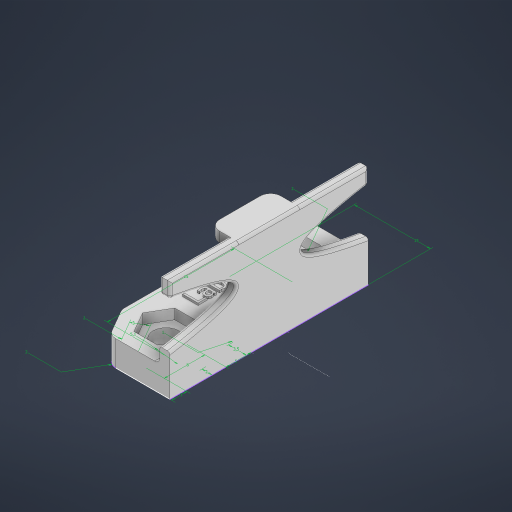
# Autodesk Inventor part: soporte_pinzas_abiertas
Saved by Autodesk Inventor 2024.1 (Build 281209000, 209)
## iProperties
Created: 2023-06-27
Part Number: soporte_pinzas_abiertas
Material: Generic
Document SubType Name: Modeling
Designer: LabTel_Admin
Density: 1 g/cm^3
Appearance: Default
Author: LabTel_Admin
Autodesk Inventor part; units mm, degrees
ref_plane "YZ Plane" through (0, 0, 0) normal (1, 0, 0) x (0, 1, 0)
ref_plane "XZ Plane" through (0, 0, 0) normal (0, 1, 0) x (-1, 0, 0)
ref_plane "XY Plane" through (0, 0, 0) normal (0, 0, 1) x (1, 0, 0)
sketch "Sketch2" plane through (0, 0, 0) normal (0, 1, 0) x (-1, 0, 0)
  line L0 (15.1065, 12.5) -> (17.4159, 16.5)
  line L1 (17.4159, 16.5) -> (22.0347, 16.5)
  line L2 (22.0347, 16.5) -> (24.3441, 12.5)
  line L3 (24.3441, 12.5) -> (22.0347, 8.5)
  line L4 (22.0347, 8.5) -> (17.4159, 8.5)
  line L5 (17.4159, 8.5) -> (15.1065, 12.5)
  circle A0 centre (19.7253, 12.5) radius 2.55
  line L6 (11.9711, 19.5) -> (22.612, 19.5)
  line L7 (24.3441, 18.5) -> (26.7031, 14.414)
  line L8 (26.9711, 13.414) -> (26.9711, 0.8204)
  line L9 (0, 0) -> (8.2774, 0) construction
  line L10 (15.1065, -12.5) -> (17.4159, -16.5)
  line L11 (17.4159, -16.5) -> (22.0347, -16.5)
  line L12 (22.0347, -16.5) -> (24.3441, -12.5)
  line L13 (24.3441, -12.5) -> (22.0347, -8.5)
  line L14 (22.0347, -8.5) -> (17.4159, -8.5)
  line L15 (17.4159, -8.5) -> (15.1065, -12.5)
  circle A1 centre (19.7253, -12.5) radius 2.55
  line L16 (13.6603, -19.5) -> (22.612, -19.5)
  line L17 (24.3441, -18.5) -> (26.7031, -14.414)
  line L18 (26.9711, -13.414) -> (26.9711, -0.8204)
  line L19 (11.9711, -19.5) -> (13.6603, -19.5)
  line L20 (26.9711, 0.8204) -> (26.9711, -0.8204)
  arc A2 (24.3441, 18.5) -> (22.612, 19.5) centre (22.612, 17.5) ccw
  arc A3 (26.9711, 13.414) -> (26.7031, 14.414) centre (24.9711, 13.414) ccw
  arc A4 (22.612, -19.5) -> (24.3441, -18.5) centre (22.612, -17.5) ccw
  arc A5 (26.7031, -14.414) -> (26.9711, -13.414) centre (24.9711, -13.414) ccw
  line L21 (11.9711, 19.5) -> (11.9711, -19.5)
  line L22 (11.9711, 3.5) -> (15.4711, 3.5)
  line L23 (15.9711, 3.366) -> (17.1876, 2.6637)
  line L24 (17.6876, 1.7976) -> (17.6876, -1.5)
  arc A6 (15.9711, 3.366) -> (15.4711, 3.5) centre (15.4711, 2.5) ccw
  arc A7 (17.6876, 1.7976) -> (17.1876, 2.6637) centre (16.6876, 1.7976) ccw
  line L25 (11.9711, -3.5) -> (15.4711, -3.5)
  line L26 (15.9711, -3.366) -> (17.1876, -2.6637)
  line L27 (17.6876, -1.7976) -> (17.6876, -1.5)
  arc A8 (15.4711, -3.5) -> (15.9711, -3.366) centre (15.4711, -2.5) ccw
  arc A9 (17.1876, -2.6637) -> (17.6876, -1.7976) centre (16.6876, -1.7976) ccw
  line L28 (13.9711, 3.5) -> (13.9711, 19.5)
  line L29 (13.9711, -3.5) -> (13.9711, -19.5)
  point P0 (19.7253, 8.5)
  point P1 (19.7253, 16.5)
  point P2 (23.7667, 19.5)
  point P3 (26.9711, 13.9499)
  point P4 (23.1894, 14.5)
  point P5 (19.7253, -8.5)
  point P6 (19.7253, -16.5)
  point P7 (23.7667, -19.5)
  point P8 (26.9711, -13.9499)
  point P9 (23.1894, -14.5)
  point P10 (25.239, 0.1796)
  point P11 (25.239, -0.1796)
  point P12 (26.9711, -7.1172)
  point P13 (13.4711, -19.5)
  dimension "d18" = 8
  dimension "d19" = 5.1
  dimension "d21" = 3
  dimension "d22" = 3
  dimension "d27" = 25
  dimension "d35" = 2
  dimension "d36" = 2
  dimension "d37" = 2
  dimension "d49" = 5
  dimension "d50" = 1
  dimension "d51" = 3.5
  dimension "d52" = 15
  dimension "d53" = 2
  constraints: 60 end point, 24 symmetric about line, 16 point on circle, 12 tangent, 11 point on line, 10 centre point, 4 midpoint, 3 horizontal, 3 vertical, 2 coincident, 2 equal radius, 2 perpendicular, 1 parallel, 16 other
  measures "d18" distance of point (19.725, 8.5) point (19.725, 16.5)
  measures "d19" diameter of A0
  measures "d21" distance between parallel lines of L6 L1
  measures "d22" distance from line of L7 point (23.189, 14.5)
  measures "d27" distance of point (19.725, -12.5) point (19.725, 12.5)
  measures "d35" radius of A2
  measures "d36" radius of A3
  measures "d37" radius of A4
  measures "d49" distance from line of L4 L22.start
  measures "d50" radius of A6
  measures "d51" distance of L22.start L22.end
  measures "d52" distance from line of L21 point (26.971, -7.117)
  measures "d53" distance between parallel lines of L21 L28
extrude "Extrusion9" add sketch "Sketch2" along normal blind 5 contours L6 L28 L22 L21 | L6 A2 L7 A3 L8 L20 L18 A5 L17 A4 L16 L29 L25 A8 L26 A9 L27 L24 A7 L23 A6 L22 L28 | L25 L29 L16 L19 L21
extrude "Extrusion10" add sketch "Sketch2" along normal blind 3 contours L0 L1 L2 L3 L4 L5 | L15 L14 L13 L12 L11 L10
extrude "Extrusion13" add sketch "Sketch2" along normal blind 20 contours L6 L28 L22 L21 | L25 L29 L16 L19 L21
extrude "Extrusion14" add sketch "Sketch2" along normal blind 18 contours L22 A6 L23 A7 L24 L27 A9 L26 A8 L25 L21
sketch "Sketch6" plane through (-13.9711, 5, 19.5) normal (-1, 0, 0) x (0, 0, 1)
  line L0 (-19.5, -5) -> (-19.5, 29.0321) construction
  line L1 (0, 0) -> (0, 15) projected
  line L2 (-5.086, 0) -> (-1, 0) projected
  line L3 (-16, 15) -> (0, 15) projected
  line L4 (-16, 0) -> (-16, 15) projected
  line L5 (-16, 7.5) -> (-13, 7.5)
  spline S0 degree 2 poles (0, 3) (-26, 7.5) (0, 12) knots 0 0 0 1 1 1
  line L6 (0, 3) -> (0, 12)
  line L7 (-39, 0) -> (-39, 15)
  spline S1 degree 2 poles (-39, 3) (-13, 7.5) (-39, 12) knots 0 0 0 1 1 1
  line L8 (-39, 3) -> (-39, 12)
  point P0 (-26, 7.5)
  dimension "d73" = 3
  dimension "d74" = 3
  dimension "d75" = 3
  constraints: 10 end point, 5 symmetric about line, 4 point on line, 1 collinear, 1 horizontal, 1 midpoint, 1 vertical, 6 other
  measures "d73" distance from line of L2 L6.start
  measures "d74" distance from line of L3 L6.end
  measures "d75" distance of L5.start L5.end
extrude "Extrusion15" cut sketch "Sketch6" against normal blind 20 contours S0 L1 | L7 S1
fillet "Fillet3" radius 1 2 edges at (-13.9711, 5, 11.5) (-13.9711, 5, -11.5)
fillet "Fillet4" radius 0.5 4 edges at (-13.9711, 12.5, 6.5) (-11.9711, 12.4968, 6.5) (-13.9711, 12.5, -6.5) (-11.9711, 12.4968, -6.5)
fillet "Fillet5" radius 0.51 14 edges at (-13.9711, 20, 11.5) (-13.8247, 17.1486, 19.5) (-12.9711, 17, 19.5) (-12.1175, 17.1486, 19.5) (-11.9711, 18.7537, 19.5) (-13.9711, 18.7537, 19.5) (-13.9711, 20, -11.5) (-11.9711, 20, 11.5) (-11.9711, 20, -11.5) (-13.8247, 17.1486, -19.5) (-12.9711, 17, -19.5) (-12.1175, 17.1486, -19.5) (-11.9711, 18.7537, -19.5) (-13.9711, 18.7537, -19.5)
sketch "Sketch7" plane through (0, 18, 0) normal (0, 1, 0) x (1, 0, 0)
  line L0 (-17.6876, 1.7976) -> (-17.6876, -1.7976) projected
  line L1 (-11.9711, -19.5) -> (-11.9711, 19.5) projected
  line L2 (-15.6876, -6) -> (-11.9711, -6)
  line L3 (-11.9711, -6) -> (-11.9711, 6)
  line L4 (-11.9711, 6) -> (-15.6876, 6)
  line L5 (-17.6876, 4) -> (-17.6876, -4)
  arc A0 (-17.6876, -4) -> (-15.6876, -6) centre (-15.6876, -4) ccw
  arc A1 (-15.6876, 6) -> (-17.6876, 4) centre (-15.6876, 4) ccw
  point P0 (0, 0)
  point P1 (-17.6876, -6)
  point P2 (-17.6876, 0)
  point P3 (-17.6876, 0)
  point P4 (-17.6876, 0)
  point P5 (-17.6876, 0)
  point P6 (-17.6876, -1.7976)
  dimension "d82" = 6
  dimension "d83" = 12
  dimension "d84" = 2
  constraints: 8 end point, 4 point on circle, 4 tangent, 3 point on line, 2 centre point, 2 coincident, 2 midpoint, 2 parallel, 1 equal radius, 1 horizontal, 1 perpendicular
  measures "d82" distance of point (-17.688, -6) point (-17.688, 0)
  measures "d83" distance of L3.end L2.end
  measures "d84" radius of A0
extrude "Extrusion16" add sketch "Sketch7" along normal blind 2
fillet "Fillet6" radius 0.5 1 edges at (-11.9711, 20, 0)
sketch "Sketch8" plane through (0, 5, 0) normal (0, 1, 0) x (1, 0, 0)
  line L0 (-23.3475, -6.083) -> (-23.3475, 6.4263) construction
  line L1 (-23.3475, 6.4263) -> (-19.8401, 6.4263) construction
  line L2 (-19.8401, 6.4263) -> (-19.8401, -6.083) construction
  line L3 (-19.8401, -6.083) -> (-23.3475, -6.083) construction
  line L4 (-26.9711, 13.414) -> (-26.9711, -13.414) projected
  line L5 (-26.9711, 0) -> (-17.8672, 0) construction
  line L6 (-17.4159, 8.5) -> (-22.0347, 8.5) projected
  line L7 (-22.0347, -8.5) -> (-17.4159, -8.5) projected
  line L8 (-20.1637, -4.0082) -> (-20.1637, -5.7742)
  line L9 (-20.1637, -5.7742) -> (-23.2117, -5.7742)
  line L10 (-23.2117, -5.7742) -> (-23.2117, -5.3692)
  line L11 (-23.2117, -5.3692) -> (-20.5243, -5.3692)
  line L12 (-20.5243, -5.3692) -> (-20.5243, -4.0082)
  line L13 (-20.5243, -4.0082) -> (-20.1637, -4.0082)
  spline S0 degree 2 poles (-20.4057, -2.4447) (-20.3712, -2.4916) (-20.2477, -2.6497) (-20.2106, -2.7238) knots 0 0 0 1 2 2 2
  spline S1 degree 2 poles (-20.2106, -2.7238) (-20.1563, -2.825) (-20.0995, -3.0152) (-20.0995, -3.1881) knots 0 0 0 1 2 2 2
  spline S2 degree 2 poles (-20.0995, -3.1881) (-20.0995, -3.3289) (-20.2057, -3.5833) (-20.302, -3.6797) knots 0 0 0 1 2 2 2
  spline S3 degree 2 poles (-20.302, -3.6797) (-20.3959, -3.7711) (-20.6725, -3.8822) (-20.8256, -3.8822) knots 0 0 0 1 2 2 2
  spline S4 degree 2 poles (-20.8256, -3.8822) (-21.0628, -3.8822) (-21.3987, -3.6821) (-21.495, -3.4648) knots 0 0 0 1 2 2 2
  spline S5 degree 2 poles (-21.495, -3.4648) (-21.5839, -3.2721) (-21.6506, -2.7485) (-21.6679, -2.4447) knots 0 0 0 1 2 2 2
  line L14 (-21.6679, -2.4447) -> (-21.742, -2.4447)
  spline S6 degree 2 poles (-21.742, -2.4447) (-21.8754, -2.4447) (-22.0409, -2.5262) (-22.0878, -2.6003) knots 0 0 0 1 2 2 2
  spline S7 degree 2 poles (-22.0878, -2.6003) (-22.1347, -2.6744) (-22.1644, -2.8868) (-22.1644, -3.0004) knots 0 0 0 1 2 2 2
  spline S8 degree 2 poles (-22.1644, -3.0004) (-22.1644, -3.1338) (-22.0853, -3.4944) (-22.0088, -3.6747) knots 0 0 0 1 2 2 2
  line L15 (-22.0088, -3.6747) -> (-22.0088, -3.697)
  line L16 (-22.0088, -3.697) -> (-22.4015, -3.697)
  spline S9 degree 2 poles (-22.4015, -3.697) (-22.4311, -3.5908) (-22.5052, -3.1931) (-22.5052, -2.9979) knots 0 0 0 1 2 2 2
  spline S10 degree 2 poles (-22.5052, -2.9979) (-22.5052, -2.7608) (-22.4311, -2.4373) (-22.3348, -2.3088) knots 0 0 0 1 2 2 2
  spline S11 degree 2 poles (-22.3348, -2.3088) (-22.241, -2.1828) (-21.9421, -2.0593) (-21.7272, -2.0593) knots 0 0 0 1 2 2 2
  line L17 (-21.7272, -2.0593) -> (-20.1637, -2.0593)
  line L18 (-20.1637, -2.0593) -> (-20.1637, -2.4447)
  line L19 (-20.1637, -2.4447) -> (-20.4057, -2.4447)
  line L20 (-20.7268, -2.4447) -> (-21.3616, -2.4447)
  spline S12 degree 2 poles (-21.3616, -2.4447) (-21.3493, -2.583) (-21.3073, -3.0004) (-21.2678, -3.1313) knots 0 0 0 1 2 2 2
  spline S13 degree 2 poles (-21.2678, -3.1313) (-21.2208, -3.2845) (-21.0257, -3.4845) (-20.8528, -3.4845) knots 0 0 0 1 2 2 2
  spline S14 degree 2 poles (-20.8528, -3.4845) (-20.6552, -3.4845) (-20.4551, -3.2622) (-20.4551, -3.0498) knots 0 0 0 1 2 2 2
  spline S15 degree 2 poles (-20.4551, -3.0498) (-20.4551, -2.8695) (-20.6107, -2.5731) (-20.7268, -2.4447) knots 0 0 0 1 2 2 2
  spline S16 degree 2 poles (-21.3443, 0.3983) (-20.7836, 0.3983) (-20.0995, -0.1451) (-20.0995, -0.5551) knots 0 0 0 1 2 2 2
  spline S17 degree 2 poles (-20.0995, -0.5551) (-20.0995, -0.7404) (-20.1908, -1.0046) (-20.2699, -1.1331) knots 0 0 0 1 2 2 2
  line L21 (-20.2699, -1.1331) -> (-20.1637, -1.1578)
  line L22 (-20.1637, -1.1578) -> (-20.1637, -1.5184)
  line L23 (-20.1637, -1.5184) -> (-23.3475, -1.5184)
  line L24 (-23.3475, -1.5184) -> (-23.3475, -1.1331)
  line L25 (-23.3475, -1.1331) -> (-22.2113, -1.1331)
  spline S18 degree 2 poles (-22.2113, -1.1331) (-22.3422, -0.9874) (-22.5151, -0.649) (-22.5151, -0.4341) knots 0 0 0 1 2 2 2
  spline S19 degree 2 poles (-22.5151, -0.4341) (-22.5151, -0.0463) (-21.8952, 0.3983) (-21.3443, 0.3983) knots 0 0 0 1 2 2 2
  spline S20 degree 2 poles (-21.3147, 0.0006) (-21.7247, 0.0006) (-22.1496, -0.2488) (-22.1496, -0.5255) knots 0 0 0 1 2 2 2
  spline S21 degree 2 poles (-22.1496, -0.5255) (-22.1496, -0.6811) (-22.0014, -1.0022) (-21.8877, -1.1331) knots 0 0 0 1 2 2 2
  line L26 (-21.8877, -1.1331) -> (-20.5762, -1.1331)
  spline S22 degree 2 poles (-20.5762, -1.1331) (-20.5045, -0.9874) (-20.4453, -0.7626) (-20.4453, -0.6292) knots 0 0 0 1 2 2 2
  spline S23 degree 2 poles (-20.4453, -0.6292) (-20.4453, -0.3353) (-20.8627, 0.0006) (-21.3147, 0.0006) knots 0 0 0 1 2 2 2
  line L27 (-20.1637, 1.5395) -> (-22.8511, 1.5395)
  line L28 (-22.8511, 1.5395) -> (-22.8511, 0.5169)
  line L29 (-22.8511, 0.5169) -> (-23.2117, 0.5169)
  line L30 (-23.2117, 0.5169) -> (-23.2117, 2.9671)
  line L31 (-23.2117, 2.9671) -> (-22.8511, 2.9671)
  line L32 (-22.8511, 2.9671) -> (-22.8511, 1.9446)
  line L33 (-22.8511, 1.9446) -> (-20.1637, 1.9446)
  line L34 (-20.1637, 1.9446) -> (-20.1637, 1.5395)
  spline S24 degree 2 poles (-20.1118, 4.2392) (-20.1118, 3.6909) (-20.7268, 3.0882) (-21.2949, 3.0882) knots 0 0 0 1 2 2 2
  spline S25 degree 2 poles (-21.2949, 3.0882) (-21.8532, 3.0882) (-22.5151, 3.6736) (-22.5151, 4.1453) knots 0 0 0 1 2 2 2
  spline S26 degree 2 poles (-22.5151, 4.1453) (-22.5151, 4.3578) (-22.3916, 4.6863) (-22.2607, 4.8073) knots 0 0 0 1 2 2 2
  spline S27 degree 2 poles (-22.2607, 4.8073) (-22.1298, 4.9308) (-21.7519, 5.0617) (-21.4777, 5.0617) knots 0 0 0 1 2 2 2
  line L35 (-21.4777, 5.0617) -> (-21.2678, 5.0617)
  line L36 (-21.2678, 5.0617) -> (-21.2678, 3.4784)
  spline S28 degree 2 poles (-21.2678, 3.4784) (-20.8701, 3.4784) (-20.4477, 3.8786) (-20.4477, 4.2343) knots 0 0 0 1 2 2 2
  spline S29 degree 2 poles (-20.4477, 4.2343) (-20.4477, 4.3602) (-20.5045, 4.6048) (-20.549, 4.7036) knots 0 0 0 1 2 2 2
  spline S30 degree 2 poles (-20.549, 4.7036) (-20.5984, 4.8073) (-20.6848, 4.9506) (-20.7244, 4.9975) knots 0 0 0 1 2 2 2
  line L37 (-20.7244, 4.9975) -> (-20.7244, 5.0197)
  line L38 (-20.7244, 5.0197) -> (-20.3045, 5.0197)
  spline S31 degree 2 poles (-20.3045, 5.0197) (-20.2773, 4.953) (-20.1983, 4.7505) (-20.176, 4.6715) knots 0 0 0 1 2 2 2
  spline S32 degree 2 poles (-20.176, 4.6715) (-20.1439, 4.5603) (-20.1118, 4.3775) (-20.1118, 4.2392) knots 0 0 0 1 2 2 2
  spline S33 degree 2 poles (-21.5617, 4.6863) (-21.7173, 4.6813) (-21.9446, 4.6171) (-22.0211, 4.5554) knots 0 0 0 1 2 2 2
  spline S34 degree 2 poles (-22.0211, 4.5554) (-22.1076, 4.4887) (-22.199, 4.2787) (-22.199, 4.1231) knots 0 0 0 1 2 2 2
  spline S35 degree 2 poles (-22.199, 4.1231) (-22.199, 3.97) (-22.1076, 3.7551) (-22.0187, 3.6662) knots 0 0 0 1 2 2 2
  spline S36 degree 2 poles (-22.0187, 3.6662) (-21.9273, 3.5797) (-21.7074, 3.4908) (-21.5617, 3.4784) knots 0 0 0 1 2 2 2
  line L39 (-21.5617, 3.4784) -> (-21.5617, 4.6863)
  line L40 (-20.1637, 5.8447) -> (-20.1637, 5.4594)
  line L41 (-20.1637, 5.4594) -> (-23.3475, 5.4594)
  line L42 (-23.3475, 5.4594) -> (-23.3475, 5.8447)
  line L43 (-23.3475, 5.8447) -> (-20.1637, 5.8447)
  point P0 (0, 0)
  point P1 (-21.5938, -6.083)
  dimension "d92" = 2.0737
  dimension "d93" = 2.417
  constraints: 2 end point, 2 midpoint, 1 horizontal, 2 other
  measures "d92" distance between parallel lines of L6 L1
  measures "d93" distance from line of L7 point (-21.594, -6.083)
extrude "Extrusion17" add sketch "Sketch8" along normal blind 0.4
body "Solid2"
